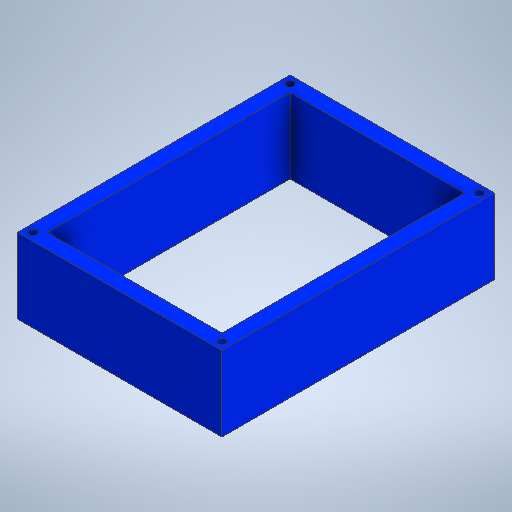
# Autodesk Inventor part: Body
Saved by Autodesk Inventor 2025.2 (Build 292293000, 293)
## iProperties
Created: 2025-01-23
Part Number: Body
Material: Generic
Document SubType Name: Modeling
Designer: User
Density: 1 g/cm^3
Appearance: Default
Author: User
Autodesk Inventor part; units mm, degrees
ref_plane "YZ Plane" through (0, 0, 0) normal (1, 0, 0) x (0, 1, 0)
ref_plane "XZ Plane" through (0, 0, 0) normal (0, 1, 0) x (-1, 0, 0)
ref_plane "XY Plane" through (0, 0, 0) normal (0, 0, 1) x (1, 0, 0)
sketch "Sketch1" plane through (0, 0, 0) normal (0, 1, 0) x (-1, 0, 0)
  line L0 (-75, 0) -> (-75, -100)
  line L1 (-75, -100) -> (75, -100)
  line L2 (75, -100) -> (75, 100)
  line L3 (75, 100) -> (-75, 100)
  line L4 (-75, 100) -> (-75, 0)
  circle A0 centre (69.3987, -94.3567) radius 3
  circle A1 centre (-69.3245, -94.3567) radius 3
  circle A2 centre (69.3987, 94.3688) radius 3
  circle A3 centre (-69.3245, 94.4539) radius 3
  line L5 (75, -100) -> (75, -97.4)
  line L6 (75, 100) -> (57, 100)
  line L7 (75, 100) -> (64, 100)
  line L8 (64, 100) -> (64, -100)
  line L9 (-75, 100) -> (-64, 100)
  line L10 (-64, 100) -> (-64, -100)
  line L11 (64, -100) -> (64, -89)
  line L12 (64, -89) -> (-64, -89)
  line L13 (64, 100) -> (64, 89)
  line L14 (64, 89) -> (-64, 89)
  point P0 (0, 0)
  dimension "d3" = 200
  dimension "d4" = 150
  dimension "d5" = 6
  dimension "d6" = 6
  dimension "d7" = 6
  dimension "d8" = 6
  dimension "d18" = 11
  constraints: 30 end point, 11 point on line, 6 perpendicular, 4 centre point
  measures "d3" distance of L1.end L2.end
  measures "d4" distance of L2.end L3.end
  measures "d5" diameter of A0
  measures "d6" diameter of A1
  measures "d7" diameter of A2
  measures "d8" diameter of A3
  measures "d18" distance of L8.end L11.end
extrude "Extrusion1" add sketch "Sketch1" along normal blind 55 contours L3 L8 L14 L10
extrude "Extrusion2" add sketch "Sketch1" along normal blind 55 contours L8 L3 L2 L1
extrude "Extrusion3" add sketch "Sketch1" along normal blind 55 contours L4 L3 L10 L1 L0
extrude "Extrusion4" add sketch "Sketch1" along normal blind 55 contours L10 L12 L8 L1
body "Solid1"
